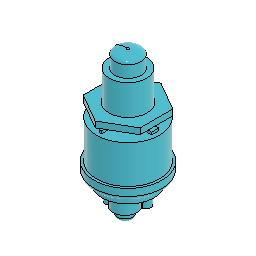
Switch 12V 50A A1 (Autodesk Fusion 360 design; units mm, degrees)
Autodesk Fusion 360 part; units mm, degrees
sketch "Sketch1" plane through (0, 0, 0) normal (0, 0, 1) x (1, 0, 0)
  circle A0 centre (0, 0) radius 5.5
  circle A1 centre (0, 0) radius 7.75
  circle A2 centre (0, 0) radius 13.25
  circle A3 centre (0, 0) radius 14.25
  line L0 (7.6035, 1.5) -> (11.5, 1.5)
  line L1 (11.5, 1.5) -> (11.5, -1.5)
  line L2 (11.5, -1.5) -> (7.6035, -1.5)
  line L3 (0.5, 7.7339) -> (0.5, 11.6304)
  line L4 (0.5, 11.6304) -> (-0.5, 11.6304)
  line L5 (-0.5, 11.6304) -> (-0.5, 7.7339)
  line L6 (-0.5, -7.7339) -> (-0.5, -11.6304)
  line L7 (-0.5, -11.6304) -> (0.5, -11.6304)
  line L8 (0.5, -11.6304) -> (0.5, -7.7339)
  line L9 (-7.7136, 0.75) -> (-11.6102, 0.75)
  line L10 (-11.6102, 0.75) -> (-11.6102, -0.75)
  line L11 (-11.6102, -0.75) -> (-7.7136, -0.75)
  point P0 (0, 11.6304)
  point P1 (11.5, 0)
  point P2 (0, -11.6304)
  point P3 (-11.6102, 0)
  dimension "d1" = 11
  dimension "d2" = 15.5
  dimension "d3" = 26.5
  dimension "d4" = 28.5
  dimension "d5" = 3
  dimension "d6" = 1
  dimension "d7" = 1.5
  dimension "d8" = 11.5
  constraint coincident A0.centre A1.centre
  constraint concentric A0 A1
  constraint concentric A1 A2
  constraint concentric A2 A3
  constraint coincident A1 L0.start
  constraint horizontal L0
  constraint perpendicular L0 L1
  constraint coincident A1 L2.end
  constraint perpendicular L1 L2
  constraint coincident A1 L3.start
  constraint perpendicular L2 L3
  constraint perpendicular L3 L4
  constraint coincident A1 L5.end
  constraint perpendicular L4 L5
  constraint coincident A1 L6.start
  constraint parallel L3 L6
  constraint perpendicular L6 L7
  constraint coincident A1 L8.end
  constraint perpendicular L7 L8
  constraint coincident A1 L9.start
  constraint perpendicular L6 L9
  constraint perpendicular L9 L10
  constraint coincident A1 L11.end
  constraint perpendicular L6 L11
  constraint midpoint L4 P0
  constraint midpoint L1 P1
  constraint midpoint L7 P2
  constraint midpoint L10 P3
  constraint vertical A0.centre P0
  constraint horizontal A0.centre P1
  constraint vertical A0.centre P2
  constraint horizontal A0.centre P3
  constraint equal L0 L3
  constraint equal L0 L8
  constraint equal L0 L9
  constraint equal L4 L7
  measures "d1" diameter of A0
  measures "d2" diameter of A1
  measures "d3" diameter of A2
  measures "d4" diameter of A3
  measures "d5" distance of L0.end L1.end
  measures "d6" distance of L3.end L4.end
  measures "d7" distance of L9.end L10.end
  measures "d8" distance of A0.centre L1
extrude "Extrude1" add sketch "Sketch1" along normal blind 5 contours A3 makes body 1
extrude "Extrude2" add sketch "Sketch1" along normal blind 21 contours A2 bodies 1
extrude "Extrude3" add sketch "Sketch1" along normal blind 22 contours A1 L0 L1 L2 | A1 L3 L4 L5 | A1 L6 L7 L8 | A1 L9 L10 L11 bodies 1
extrude "Extrude4" add sketch "Sketch1" along normal blind 39 contours A1 bodies 1
extrude "Extrude5" add sketch "Sketch1" along normal blind 46 contours A0 bodies 1
sketch "Sketch2" plane through (0, 0, 0) normal (0, 0, 1) x (1, 0, 0)
  circle A0 centre (0, 0) radius 11
  line L0 (0, 0) -> (11, 0) construction
  line L1 (0, 0) -> (6.3093, -9.0107) construction
  circle A1 centre (2.8679, -4.0958) radius 5
  circle A2 centre (2.8679, -4.0958) radius 3.25
  circle A3 centre (2.8679, -4.0958) radius 4
  line L2 (0, 0) -> (9.0107, 6.3093) construction
  circle A4 centre (4.5053, 3.1547) radius 2
  arc A5 (4.8894, 1.1919) -> (0.2447, -1.076) centre (6.8124, -8.6366) ccw
  line L3 (0.5661, -0.8084) -> (0, 0)
  line L4 (0, 0) -> (-0.5661, 0.8084)
  arc A6 (-0.5661, 0.8084) -> (2.7923, 4.1869) centre (-5.7858, 9.3555) ccw
  circle A7 centre (-2.8679, 4.0958) radius 5
  circle A8 centre (-2.8679, 4.0958) radius 3.25
  line L5 (6.9636, -1.2279) -> (1.2279, 6.9636)
  line L6 (-1.2279, -6.9636) -> (-6.9636, 1.2279)
  dimension "d19" = 22
  dimension "d20" = 55
  dimension "d21" = 10
  dimension "d22" = 6.5
  dimension "d23" = 8
  dimension "d24" = 4
  dimension "d25" = 5.5
  dimension "d27" = 10
  dimension "d31" = 6.5
  constraint coincident A0.centre L0.start
  constraint coincident A0 L0.end
  constraint horizontal L0
  constraint coincident A0 L1.end
  constraint coincident L1 A1.centre
  constraint coincident A0.centre A1
  constraint concentric A1 A2
  constraint concentric A1 A3
  constraint coincident A0 L2.end
  constraint perpendicular L1 L2
  constraint coincident L2 A4.centre
  constraint coincident A3 A5.end
  constraint coincident A4 A5.start
  constraint tangent A3 A5
  constraint tangent A4 A5
  constraint coincident A5 L3.start
  constraint coincident L1 L3.start
  constraint perpendicular L2 L4
  constraint equal L3 L4
  constraint coincident A0 A5.centre
  constraint coincident A4 A6.end
  constraint coincident A0 A6.centre
  constraint coincident L4.end A6.start
  constraint tangent A4 A6
  constraint coincident L1 A7.centre
  constraint coincident A0.centre A7
  constraint coincident A1 L5.start
  constraint coincident A7 L5.end
  constraint coincident A1 L6.start
  constraint coincident A7 L6.end
  constraint tangent A7 L6
  constraint tangent A1 L6
  constraint tangent A7 L5
  constraint tangent A1 L5
  constraint coincident A7.centre A8.centre
  measures "d19" diameter of A0
  measures "d20" angle of L0 L1
  measures "d21" diameter of A1
  measures "d22" diameter of A2
  measures "d23" diameter of A3
  measures "d24" diameter of A4
  measures "d25" distance of A0.centre A4.centre
  measures "d27" diameter of A7
  measures "d31" diameter of A8
extrude "Extrude6" add sketch "Sketch2" against normal blind 3 contours A0 | A1 A4 A5 L5 | A1 A7 L6 | A1 A4 A5 A6 A7 | L4 A6 A7 | A4 A6 A7 L5 picked at (0.1045, 0.8903) bodies 1
extrude "Extrude7" add sketch "Sketch2" against normal blind 8 contours A1 A5 L3 | A1 A4 A5 L5 | A1 A7 L6 | A1 A5 L3 | A1 A4 A5 A6 A7 | A4 L5 | L4 A6 A7 | L4 A6 A7 | A4 A6 A7 L5 | A2 | A3 | A8 picked at (3.6, 2.7521) bodies 1
extrude "Extrude8" add sketch "Sketch2" against normal blind 10.5 contours A1 A5 L3 | A1 A4 A5 A6 A7 | A4 L5 | A4 L5 | L4 A6 A7 picked at (0.8724, -0.2063) picked at (0.1045, 0.8903) bodies 1
pattern_circular "C-Pattern1" count 2 over 360 about axis through (0, 0, 0) along (0, 0, -1) of "Extrude8"
extrude "Extrude9" add sketch "Sketch2" against normal blind 12 contours A2 | A8 bodies 1
fillet "Fillet1" radius 2 1 edges at (-13.2857, -5.153, 0) on bodies 1
fillet "Fillet2" radius 1.5 2 edges at (-5.8979, 5.271, -12) (-0.1622, -2.9205, -12) on bodies 1
fillet "Fillet3" offset 5 second offset 2 1 edges at (-5.1278, -1.9889, 46) measured on face at (-1.4907, 0.2732, 46) on bodies 1
sketch "Sketch3" plane through (0, 0, 0) normal (0, 0, 1) x (1, 0, 0)
  line L0 (-12, -6.9282) -> (0, -13.8564)
  line L1 (0, -13.8564) -> (12, -6.9282)
  line L2 (12, -6.9282) -> (12, 6.9282)
  line L3 (12, 6.9282) -> (0, 13.8564)
  line L4 (0, 13.8564) -> (-12, 6.9282)
  line L5 (-12, 6.9282) -> (-12, -6.9282)
  circle A0 centre (0, 0) radius 8
  dimension "d47" = 12
  dimension "d51" = 16
  constraint coincident A0.centre origin
  constraint vertical L5
  measures "d47" distance of A0.centre L5
  measures "d51" diameter of A0
extrude "Extrude10" add sketch "Sketch3" along normal blind 2.5 from surface at 24 separate body makes body 2
equation "d8 = ( 23 / 2 ) * 1 mm"
equation "d25 = ( 11 / 2 ) * 1 mm"
equation "d47 = ( 24 / 2 ) * 1 mm"
